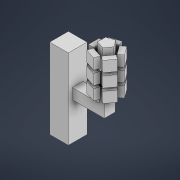
# Autodesk Inventor part: 110033226_ipt_38_小河方塊
Saved by Autodesk Inventor 2022 (Build 260153000, 153)
## iProperties
Created: 2022-06-25
Part Number: 110033226_ipt_38_小河方塊
Material: 一般
Document SubType Name: Modeling
Designer: User
Density: 1 g/cm^3
Appearance: 預設
Author: User
Autodesk Inventor part; units mm, degrees
ref_plane "YZ Plane" through (0, 0, 0) normal (1, 0, 0) x (0, 1, 0)
ref_plane "XZ Plane" through (0, 0, 0) normal (0, 1, 0) x (-1, 0, 0)
ref_plane "XY Plane" through (0, 0, 0) normal (0, 0, 1) x (1, 0, 0)
sketch "草圖1" plane through (0, 0, 0) normal (0, 1, 0) x (-1, 0, 0)
  line L0 (0, 0) -> (5, 0)
  line L1 (5, 0) -> (5, -25)
  line L2 (5, -25) -> (0, -25)
  line L3 (0, -25) -> (0, 0)
  circle A0 centre (2.5, -2.5) radius 1.7
  line L4 (4.25, -0.75) -> (0.75, -0.75)
  line L5 (0.75, -0.75) -> (0.75, -4.25)
  line L6 (0.75, -4.25) -> (4.25, -4.25)
  line L7 (4.25, -4.25) -> (4.25, -0.75)
  point P0 (4.25, -2.5)
  point P1 (2.5, -4.25)
  dimension "d0" = 5
  dimension "d1" = 25
  dimension "d2" = 3.4
  dimension "d3" = 2.5
  dimension "d4" = 2.5
  dimension "d5" = 3.5
  dimension "d6" = 3.5
  constraints: 16 end point, 4 parallel, 2 horizontal, 2 midpoint, 2 perpendicular, 1 centre point, 1 horizontal alignment, 1 vertical alignment
  measures "d0" distance of L1.end L2.end
  measures "d1" distance of L0.end L1.end
  measures "d2" diameter of A0
  measures "d3" distance from line of L3 A0.centre
  measures "d4" distance from line of L0 A0.centre
  measures "d5" distance of L6.end L5.end
  measures "d6" distance of L5.end L4.end
extrude "擠出1" add sketch "草圖1" along normal blind 15 contours A0 | L7 L6 L5 L4
sketch "草圖2" plane through (-0.75, 0, -0.75) normal (1, 0, 0) x (0, 0, -1)
  line L0 (3.5, 15) -> (3.5, 0) projected
  line L1 (3.5, 0) -> (0, 0) projected
  line L2 (0, 0) -> (0, 15) projected
  line L3 (0, 15) -> (3.5, 15) projected
  line L4 (3.5, 15) -> (3.5, 0) projected
  line L5 (3.5, 0) -> (0, 0) projected
  line L6 (0, 0) -> (0, 15) projected
  line L7 (0, 15) -> (3.5, 15) projected
  line L8 (0, 0) -> (0, 15) projected
  line L9 (0, 10) -> (4, 10)
  line L10 (4, 10) -> (4, 6)
  line L11 (4, 6) -> (0, 6)
  line L12 (0, 6) -> (0, 10)
  line L13 (3.5, 0) -> (3.5, 15) projected
  line L14 (3.5, 10) -> (3.5, 6)
  line L15 (0.75, 9) -> (2.75, 9)
  line L16 (2.75, 9) -> (2.75, 7)
  line L17 (2.75, 7) -> (0.75, 7)
  line L18 (0.75, 7) -> (0.75, 9)
  point P0 (-0.75, 0)
  point P1 (1.75, 9)
  point P2 (1.75, 15)
  point P3 (2.75, 8)
  point P4 (4, 8)
  dimension "d9" = 4
  dimension "d10" = 4
  dimension "d11" = 5
  dimension "d12" = 2
  dimension "d13" = 2
  constraints: 18 end point, 5 point on line, 4 midpoint, 4 parallel, 2 horizontal, 2 perpendicular, 1 horizontal alignment, 1 vertical alignment
  measures "d9" distance of L10.end L11.end
  measures "d10" distance of L9.end L10.end
  measures "d11" distance between parallel lines of L3 L9
  measures "d12" distance of L16.end L17.end
  measures "d13" distance of L15.end L16.end
extrude "擠出2" add sketch "草圖2" along normal blind 6 contours L15 L16 L17 L18
sketch "草圖3" plane through (-0.75, 9, -1.5) normal (0, 1, 0) x (1, 0, 0)
  line L0 (0, -0.75) -> (-3.5, -0.75) projected
  line L1 (-3.5, -0.75) -> (-3.5, 2.75) projected
  line L2 (-3.5, 2.75) -> (0, 2.75) projected
  line L3 (0, 2.75) -> (0, 2) projected
  line L4 (0, 2) -> (0, 0) projected
  line L5 (0, 0) -> (0, -0.75) projected
  line L6 (0, 2) -> (6, 2) projected
  line L7 (6, 2) -> (6, 0) projected
  line L8 (6, 0) -> (0, 0) projected
  line L9 (6, 0) -> (5, 0)
  line L10 (5, 0) -> (5, 2)
  line L11 (5, 2) -> (6, 2)
  line L12 (6, 2) -> (6, 0)
  point P0 (0.75, -1.5)
  point P1 (5, 0)
  dimension "d16" = 1
  dimension "d17" = 2
  constraints: 8 end point, 2 parallel, 1 horizontal, 1 perpendicular
  measures "d16" distance of L10.end L11.end
  measures "d17" distance of L9.end L10.end
extrude "擠出3" add sketch "草圖3" along normal blind 5 contours L10 L6 L7 L8
sketch "草圖4" plane through (-0.75, 14, -1.5) normal (0, 1, 0) x (1, 0, 0)
  line L0 (4, 0) -> (3, 0)
  line L1 (3, 0) -> (3, 2)
  line L2 (3, 2) -> (4, 2)
  line L3 (4, 2) -> (4, 0)
  line L4 (5, 2) -> (5, 0) projected
  point P0 (0.75, -1.5)
  point P1 (4, 1)
  point P2 (5, 1)
  dimension "d20" = 1
  dimension "d21" = 2
  dimension "d22" = 1
  constraints: 8 end point, 2 midpoint, 2 parallel, 1 horizontal, 1 horizontal alignment, 1 perpendicular
  measures "d20" distance of L1.end L2.end
  measures "d21" distance of L0.end L1.end
  measures "d22" distance between parallel lines of L4 L3
extrude "擠出4" add sketch "草圖4" along normal mid plane 2
ref_plane "工作平面1" through (-0.75, 7, -2.5) normal (0, 0, -1) x (-1, 0, 0)
pattern_circular "環形陣列1" count 5 over 360 about axis through (4.75, 9, -2.5) along (0, -1, 0) of "擠出4"
pattern_linear "矩形陣列1" count 3 spacing 2.5 along (0, 1, 0) of "擠出4", "環形陣列1" first direction both ways yes
sketch "草圖5" plane through (2.25, 17.5, -3.5) normal (0, 1, 0) x (1, 0, 0)
  line L0 (2, -2) -> (3, -2) projected
  line L1 (3, -2) -> (3, 0) projected
  line L2 (3, 0) -> (2, 0) projected
  line L3 (2, 0) -> (2, -2) projected
  line L4 (1.447, -0.2211) -> (2.8941, 0.2491)
  line L5 (2.8941, 0.2491) -> (3.7885, -0.9819)
  line L6 (3.7885, -0.9819) -> (2.8941, -2.2129)
  line L7 (2.8941, -2.2129) -> (1.447, -1.7427)
  line L8 (1.447, -1.7427) -> (1.447, -0.2211)
  line L9 (4.3013, -1.0727) -> (3.1257, -2.6907) projected
  line L10 (2.4941, -0.9819) -> (2.0365, 0.4266) construction
  line L11 (2.9875, 0.7356) -> (1.0854, 0.1176) construction
  line L12 (1.0854, 0.1176) -> (2.9875, 0.7356) construction
  point P0 (-2.25, -3.5)
  point P1 (2.2388, -2)
  point P2 (2.8717, -2)
  point P3 (2, -1.9224)
  point P4 (2, -0.0414)
  point P5 (2.1275, 0)
  constraints: 12 end point, 1 midpoint, 1 parallel, 1 perpendicular, 11 other
extrude "擠出5" add sketch "草圖5" along normal mid plane 2 contours L7 L3 L4 L2 L1 L0 | L0 L1 L2 L4 L5 L6 L7 | L7 L8 L4 L3
